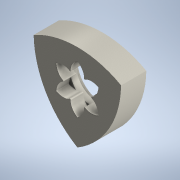
# Autodesk Inventor part: Rotor_Geared_6t_Mountable
Saved by Autodesk Inventor 2021 (Build 250183000, 183)
## iProperties
Created: 2021-03-24
Part Number: Rotor_Geared_6t_Mountable
Material: Stainless Steel
Document SubType Name: Modeling
Designer: lucia
Density: 8 g/cm^3
Appearance: Steel - Cast
Mass: 6399.98 g
Surface Area: 815.335 cm^2
Volume: 799.997 cm^3
Author: lucia
Autodesk Inventor part; units mm, degrees
ref_plane "YZ Plane" through (0, 0, 0) normal (1, 0, 0) x (0, 1, 0)
ref_plane "XZ Plane" through (0, 0, 0) normal (0, 1, 0) x (-1, 0, 0)
ref_plane "XY Plane" through (0, 0, 0) normal (0, 0, 1) x (1, 0, 0)
sketch "Sketch1" plane through (0, 0, 0) normal (0, 0, 1) x (1, 0, 0)
  line L0 (0.0008, -101.6013) -> (87.9885, 50.7987)
  line L1 (0.0008, -101.6013) -> (-87.9879, 50.7987)
  line L2 (87.9885, 50.7987) -> (-87.9879, 50.7987)
  line L3 (0.0019, 75.1827) -> (0.0019, 73.5952)
  arc A0 (87.9885, 50.7987) -> (-87.9879, 50.7987) centre (0.0003, -107.6081) ccw
  arc A1 (0.0008, -101.6013) -> (87.9885, 50.7987) centre (-93.1899, 53.8017) ccw
  arc A2 (-87.9879, 50.7987) -> (0.0008, -101.6013) centre (93.1905, 53.8024) ccw
  circle A3 centre (0, 0) radius 39.624
  point P0 (114.808, -13.208)
  dimension "d3" = 60
  dimension "d4" = 1.5875
  dimension "d5" = 79.248
  constraints: 8 end point, 7 point on circle, 4 centre point, 2 equal radius, 1 coincident, 1 horizontal, 1 vertical, 6 other
  measures "d3" angle of L1 L0
  measures "d4" distance of L3.start L3.end
  measures "d5" diameter of A3
extrude "Extrusion1" add sketch "Sketch1" against normal blind 50.8
sketch "Sketch2" plane through (0, 0, 0) normal (0, 0, 1) x (1, 0, 0)
  circle A0 centre (0, 0) radius 28.0184
  circle A1 centre (0, 0) radius 39.624
  dimension "d118" = 56.0368
  dimension "d119" = 79.248
  constraints: 2 centre point, 2 coincident
  measures "d118" diameter of A0
  measures "d119" diameter of A1
extrude "Extrusion2" add sketch "Sketch2" against normal blind 25.4
sketch "Sketch3" plane through (0, 0, 0) normal (0, 0, 1) x (1, 0, 0)
  circle A0 centre (0, 0) radius 39.624
  circle A1 centre (0, 0) radius 26.416
  circle A2 centre (0, 0) radius 28.0184
  circle A3 centre (0, 0) radius 52.832
  line L0 (0, 0) -> (12.8557, 24.895)
  line L1 (0, 0) -> (10.7834, 25.8602)
  line L2 (0, 0) -> (8.6394, 26.6532)
  line L3 (0, 0) -> (6.4378, 27.2688)
  line L4 (0, 0) -> (4.1934, 27.7028)
  line L5 (0, 0) -> (1.9211, 27.9525)
  line L6 (0, 0) -> (-0.364, 28.016)
  line L7 (0, 0) -> (-2.6467, 27.8931)
  line L8 (0, 0) -> (-4.9118, 27.5845)
  line L9 (0, 0) -> (-7.1442, 27.0923)
  line L10 (12.8557, 24.895) -> (10.7834, 25.8602)
  line L11 (10.7834, 25.8602) -> (8.6394, 26.6532)
  line L12 (8.6394, 26.6532) -> (6.4378, 27.2688)
  line L13 (6.4378, 27.2688) -> (4.1934, 27.7028)
  line L14 (4.1934, 27.7028) -> (1.9211, 27.9525)
  line L15 (1.9211, 27.9525) -> (-0.364, 28.016)
  line L16 (-0.364, 28.016) -> (-2.6467, 27.8931)
  line L17 (-2.6467, 27.8931) -> (-4.9118, 27.5845)
  line L18 (-4.9118, 27.5845) -> (-7.1442, 27.0923)
  line L19 (0, 0) -> (0, 57.682)
  circle A4 centre (0, 0) radius 39.624 projected
  line L20 (10.7834, 25.8602) -> (12.8934, 24.9804)
  line L21 (8.6394, 26.6532) -> (12.9886, 25.2434)
  line L22 (6.4378, 27.2688) -> (13.1123, 25.693)
  line L23 (4.1934, 27.7028) -> (13.2344, 26.3343)
  line L24 (1.9211, 27.9525) -> (13.3242, 27.1688)
  line L25 (-0.364, 28.016) -> (13.3508, 28.1942)
  line L26 (-2.6467, 27.8931) -> (13.2837, 29.4047)
  line L27 (-4.9118, 27.5845) -> (13.093, 30.7905)
  line L28 (-7.1442, 27.0923) -> (12.7498, 32.3383)
  line L29 (0, 0) -> (-9.329, 26.4197)
  line L30 (0, 0) -> (-11.4517, 25.5713)
  line L31 (0, 0) -> (-13.4982, 24.5526)
  line L32 (0, 0) -> (-15.4548, 23.3705)
  line L33 (0, 0) -> (-17.3086, 22.0328)
  line L34 (0, 0) -> (-19.0471, 20.5484)
  line L35 (-7.1442, 27.0923) -> (-9.329, 26.4197)
  line L36 (-9.329, 26.4197) -> (-11.4517, 25.5713)
  line L37 (-11.4517, 25.5713) -> (-13.4982, 24.5526)
  line L38 (-13.4982, 24.5526) -> (-15.4548, 23.3705)
  line L39 (-15.4548, 23.3705) -> (-17.3086, 22.0328)
  line L40 (-17.3086, 22.0328) -> (-19.0471, 20.5484)
  line L41 (-9.329, 26.4197) -> (12.2267, 34.0312)
  line L42 (-11.4517, 25.5713) -> (11.498, 35.849)
  line L43 (-13.4982, 24.5526) -> (10.5405, 37.7683)
  line L44 (-15.4548, 23.3705) -> (9.3333, 39.7628)
  line L45 (-17.3086, 22.0328) -> (7.8584, 41.8035)
  line L46 (-19.0471, 20.5484) -> (6.1009, 43.859)
  line L47 (0, 0) -> (-20.6588, 18.9273)
  line L48 (0, 0) -> (-22.1331, 17.1802)
  line L49 (0, 0) -> (-23.4599, 15.3187)
  line L50 (0, 0) -> (-24.6307, 13.3552)
  line L51 (-19.0471, 20.5484) -> (-20.6588, 18.9273)
  line L52 (-20.6588, 18.9273) -> (-22.1331, 17.1802)
  line L53 (-22.1331, 17.1802) -> (-23.4599, 15.3187)
  line L54 (-23.4599, 15.3187) -> (-24.6307, 13.3552)
  line L55 (-20.6588, 18.9273) -> (4.0494, 45.8959)
  line L56 (-22.1331, 17.1802) -> (1.6961, 47.8791)
  line L57 (-23.4599, 15.3187) -> (-0.9629, 49.7721)
  line L58 (-24.6307, 13.3552) -> (-3.9275, 51.5375)
  spline S0 degree 4 poles (12.8557, 24.895) (12.8817, 24.9459) (12.9881, 25.2045) (13.1179, 25.6562) (13.2623, 26.4356) (13.3456, 27.2671) (13.3682, 28.2944) (13.2959, 29.505) (13.1003, 30.8919) (12.7519, 32.4404) (12.2236, 34.1341) (11.4896, 35.9525) (10.5265, 37.8722) (9.3136, 39.8669) (7.8328, 41.9076) (6.0692, 43.9628) (3.183, 46.8191) (0.3783, 48.9859) (-2.059, 50.5248) (-3.9275, 51.5375) knots 0 0 0 0 0 0.052182 0.082932 0.11875 0.158948 0.203072 0.250788 0.301837 0.356012 0.413138 0.473069 0.535678 0.600854 0.668498 0.738525 0.810854 1 1 1 1 1
  line L59 (10.2554, 38.2738) -> (0, 0)
  spline S1 degree 4 poles (-12.8557, 24.895) (-12.8817, 24.9459) (-12.9881, 25.2045) (-13.1179, 25.6562) (-13.2623, 26.4356) (-13.3456, 27.2671) (-13.3682, 28.2944) (-13.2959, 29.505) (-13.1003, 30.8919) (-12.7519, 32.4404) (-12.2236, 34.1341) (-11.4896, 35.9525) (-10.5265, 37.8722) (-9.3136, 39.8669) (-7.8328, 41.9076) (-6.0692, 43.9628) (-3.183, 46.8191) (-0.3783, 48.9859) (2.059, 50.5248) (3.9275, 51.5375) knots 0 0 0 0 0 0.052182 0.082932 0.11875 0.158948 0.203072 0.250788 0.301837 0.356012 0.413138 0.473069 0.535678 0.600854 0.668498 0.738525 0.810854 1 1 1 1 1
  circle A5 centre (0, 0) radius 45.6438
  line L60 (0, 0) -> (14.0092, 24.2646)
  circle A6 centre (0, 0) radius 28.0184 projected
  line L61 (13.2344, 26.3343) -> (13.2344, 26.3341)
  line L62 (0, 0) -> (-14.0092, 24.2646)
  line L63 (13.2344, 26.3343) -> (14.2789, 26.3343)
  line L64 (14.0092, 24.2646) -> (13.01, 24.8415) construction
  line L65 (13.01, 24.8415) -> (13.2344, 26.3343) construction
  spline S2 degree 2 poles (14.0092, 24.2646) (13.01, 24.8415) (13.2344, 26.3343) knots 1 1 1 2 2 2
  line L66 (-14.0092, 24.2646) -> (-13.01, 24.8415) construction
  line L67 (-13.01, 24.8415) -> (-13.2344, 26.3343) construction
  spline S3 degree 2 poles (-14.0092, 24.2646) (-13.01, 24.8415) (-13.2344, 26.3343) knots 1 1 1 2 2 2
  arc A7 (0.3274, 48.8943) -> (0, 48.8954) centre (0, 0) ccw
  line L68 (0, 48.8954) -> (0, 49.124)
  arc A8 (0, 48.8954) -> (-0.3274, 48.8943) centre (0, 0) ccw
  point P0 (-12.8934, 24.9804)
  point P1 (-12.9886, 25.2434)
  point P2 (-13.1123, 25.693)
  point P3 (-13.3242, 27.1688)
  point P4 (-13.3508, 28.1942)
  point P5 (-13.2837, 29.4047)
  point P6 (-13.093, 30.7905)
  point P7 (-12.7498, 32.3383)
  point P8 (-12.2267, 34.0312)
  point P9 (-11.498, 35.849)
  point P10 (-10.5405, 37.7683)
  point P11 (-9.3333, 39.7628)
  point P12 (-7.8584, 41.8035)
  point P13 (-6.1009, 43.859)
  point P14 (-4.0494, 45.8959)
  point P15 (-1.6961, 47.8791)
  point P16 (0.9629, 49.7721)
  point P17 (0, 49.124)
  point P18 (-12.8557, 24.895)
  point P19 (4.5644, 45.415)
  point P20 (-4.5644, 45.415)
  point P21 (-0.3274, 48.8943)
  dimension "d87" = 56.0368
  dimension "d84" = 105.664
  dimension "d85" = 79.248
  dimension "d86" = 52.832
  dimension "d88" = 2.286
  dimension "d149" = 2.286
  dimension "d150" = 4.572
  dimension "d151" = 6.858
  dimension "d152" = 9.144
  dimension "d153" = 11.43
  dimension "d154" = 13.716
  dimension "d155" = 16.002
  dimension "d156" = 18.288
  dimension "d157" = 20.574
  dimension "d158" = 22.86
  dimension "d159" = 25.146
  dimension "d160" = 27.432
  dimension "d161" = 29.718
  dimension "d162" = 32.004
  dimension "d163" = 34.29
  dimension "d164" = 36.576
  dimension "d165" = 38.862
  dimension "d166" = 41.148
  dimension "d167" = 43.434
  dimension "d168" = 15
  dimension "d169" = 91.2876
  dimension "d170" = 30
  dimension "d172" = 30
  dimension "d175" = 0.2286
  constraints: 130 end point, 22 symmetric about line, 18 equal length, 7 coincident, 6 centre point, 4 point on circle, 1 horizontal, 1 perpendicular, 1 point on line, 1 vertical, 99 other
  measures "d84" diameter of A3
  measures "d85" diameter of A0
  measures "d86" diameter of A1
  measures "d88" distance of L0.end L1.end
  measures "d149" distance of L1.end L20.end
  measures "d150" distance of L2.end L21.end
  measures "d151" distance of L3.end L22.end
  measures "d152" distance of L4.end L23.end
  measures "d153" distance of L5.end L24.end
  measures "d154" distance of L6.end L25.end
  measures "d155" distance of L7.end L26.end
  measures "d156" distance of L8.end L27.end
  measures "d157" distance of L9.end L28.end
  measures "d158" distance of L29.end L41.end
  measures "d159" distance of L30.end L42.end
  measures "d160" distance of L31.end L43.end
  measures "d161" distance of L32.end L44.end
  measures "d162" distance of L33.end L45.end
  measures "d163" distance of L34.end L46.end
  measures "d164" distance of L47.end L55.end
  measures "d165" distance of L48.end L56.end
  measures "d166" distance of L49.end L57.end
  measures "d167" distance of L50.end L58.end
  measures "d168" angle of L19 L59
  measures "d169" diameter of A5
  measures "d170" angle of L19 L60
  measures "d172" angle of L19 L62
  measures "d175" distance of L68.start L68.end
extrude "Extrusion3" cut sketch "Sketch3" against normal blind 25.4 contours L59 L43 L19 L44 A0 | A0 L44 S0 | S0 L43 L59 | L44 L19 L45 A0 | A0 L45 S0 L44 | S0 L42 L59 L43 | L59 L42 L19 L43 | S1 A5 L57 A0 | A0 L57 S1 | L45 L19 L46 A0 | A0 L46 S0 L45 | L44 S1 L45 L19 | L19 L43 S1 L44 | S0 L41 L59 L42 | L19 L42 A2 S1 L43 | L59 L41 L19 L42 | L57 A5 L56 A0 | A0 L56 S1 L57 | S1 L57 A5 | L46 L19 A0 | A0 L19 L55 A5 S0 L46 | L45 S1 L46 L19 | S1 L43 A2 S3 L44 | L44 S3 L45 S1 | S0 L28 L59 L41 | L19 L41 A2 L42 | S1 A2 L43 | L59 L28 L19 L41 | L56 A5 L19 L55 A0 | A0 L55 S1 L56 | L57 S1 A8 L19 L56 A5 | A2 S0 S2 | A5 L55 S0 | L19 L46 S1 L55 A0 | A0 L55 L19 | L45 S3 L46 S1 | S0 L27 L59 L28 | L19 L28 A2 L41 | L59 L27 L19 L28 | L56 L19 A5 | A2 L20 S0 | S0 L22 L59 L23 | L23 L59 L24 S0 | L55 A5 L19 L56 S0 | L55 L19 A5 | L46 S3 S1 | S0 L26 L59 L27 | L19 L27 A2 L28 | L59 L26 L19 L27 | L19 A7 S0 L56 | A2 L21 S0 L20 | L59 L22 A2 L23 | L23 A2 L24 L59 | S0 L21 A2 L59 L22 | L24 L59 L25 S0 | L22 L59 A2 | A2 L25 L59 L24 | A2 L26 L19 | A2 L27 L19 L26 | S0 L25 L59 L26 | L59 L25 L19 L26
pattern_circular "Circular Pattern1" count 6 over 360 about axis through (0, 0, 0) along (0, 0, -1) of "Extrusion3"
sketch "Sketch11" plane through (0, 0, -50.8) normal (0, 0, -1) x (-1, 0, 0)
  circle A0 centre (0, 0) radius 39.624
  circle A1 centre (0, 0) radius 50.8
  line L0 (0, 0) -> (0, 50.8)
  circle A2 centre (0, 0) radius 39.624 projected
  line L1 (0, 0) -> (25.4, 43.9941)
  line L2 (-50.8, 0) -> (50.8, 0)
  line L3 (0, 0) -> (-25.4, 43.9941)
  line L4 (0, 0) -> (25.4, -43.9941)
  line L5 (0, 0) -> (-25.4, -43.9941)
  circle A3 centre (22.606, 39.1547) radius 2.7781
  circle A4 centre (45.212, 0) radius 2.7781
  circle A5 centre (-22.606, 39.1547) radius 2.7781
  circle A6 centre (-45.212, 0) radius 2.7781
  circle A7 centre (22.606, -39.1547) radius 2.7781
  circle A8 centre (-22.606, -39.1547) radius 2.7781
  dimension "d182" = 79.248
  dimension "d183" = 101.6
  dimension "d192" = 30
  dimension "d194" = 45.212
  dimension "d195" = 45.212
  dimension "d196" = 5.5563
  dimension "d197" = 5.5563
  constraints: 12 end point, 8 centre point, 7 symmetric about line, 4 point on circle, 2 coincident, 2 point on line, 1 horizontal, 1 midpoint, 1 vertical, 4 other
  measures "d182" diameter of A0
  measures "d183" diameter of A1
  measures "d192" angle of L0 L1
  measures "d194" distance of point (0, 0) A3.centre
  measures "d195" distance of point (0, 0) A4.centre
  measures "d196" diameter of A4
  measures "d197" diameter of A3
extrude "Extrusion7" cut sketch "Sketch11" against normal blind 12.7 contours L2 A4 A1 L4 A7 A0 | A0 L1 A3 A1 L2 A4 | A0 L0 A1 L1 A3 | L4 A7 A1 L5 A8 A0 | A4 L2 | L2 A4 | A0 L3 A5 A1 L0 | A3 L1 | L1 A3 | L5 A8 A1 L2 A6 A0 | A7 L4 | L4 A7 | L2 A6 A1 L3 A5 A0 | A8 L5 | L5 A8 | A6 L2 | L2 A6 | A5 L3 | L3 A5
sketch "Sketch12" plane through (0, 0, -38.1) normal (0, 0, -1) x (-1, 0, 0)
  circle A0 centre (0, 0) radius 39.624
  circle A1 centre (0, 0) radius 50.8
  line L0 (0, 0) -> (0, 50.8)
  circle A2 centre (0, 0) radius 39.624
  line L1 (0, 0) -> (25.4, 43.9941)
  line L2 (-50.8, 0) -> (50.8, 0)
  line L3 (0, 0) -> (-25.4, 43.9941)
  line L4 (0, 0) -> (25.4, -43.9941)
  line L5 (0, 0) -> (-25.4, -43.9941)
  circle A3 centre (22.606, 39.1547) radius 2.7781
  circle A4 centre (45.212, 0) radius 2.7781
  circle A5 centre (-22.606, 39.1547) radius 2.7781
  circle A6 centre (-45.212, 0) radius 2.7781
  circle A7 centre (22.606, -39.1547) radius 2.7781
  circle A8 centre (-22.606, -39.1547) radius 2.7781
  dimension "d198" = 79.248
  dimension "d199" = 101.6
  dimension "d200" = 30
  dimension "d201" = 45.212
  dimension "d202" = 45.212
  dimension "d203" = 5.5563
  dimension "d204" = 5.5563
  constraints: 12 end point, 9 centre point, 7 symmetric about line, 4 point on circle, 2 coincident, 2 point on line, 1 horizontal, 1 midpoint, 1 vertical, 4 other
  measures "d198" diameter of A0
  measures "d199" diameter of A1
  measures "d200" angle of L0 L1
  measures "d201" distance of point (0, 0) A3.centre
  measures "d202" distance of point (0, 0) A4.centre
  measures "d203" diameter of A4
  measures "d204" diameter of A3
extrude "Extrusion8" cut sketch "Sketch12" against normal blind 25.4 contours A4 L2 | L2 A4 | A3 L1 | L1 A3 | A7 L4 | L4 A7 | A8 L5 | L5 A8 | A6 L2 | L2 A6 | A5 L3 | L3 A5
equation "\"prcsn\" = 0.5715"
equation "\"d45\" = 0.5842"
equation "\"d64\" = 0.5842"
equation "\"d83\" = 0.5842"
equation "\"d115\" = 0.7112"
equation "\"d138\" = 0.7112"
equation "\"radius\" = 3.81"
body "Solid1"
